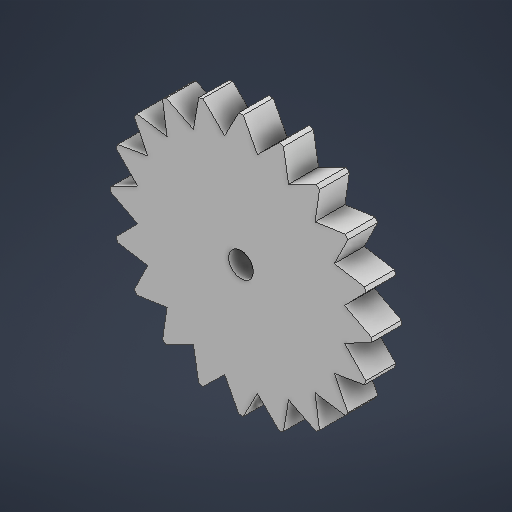
# Autodesk Inventor part: Gear_Basic
Saved by Autodesk Inventor 2026.1 (Build 301233020, 233B)
## iProperties
Created: 2026-03-11
Part Number: Gear_Basic
Material: Generic
Document SubType Name: Modeling
Designer: elaij
Density: 1 g/cm^3
Appearance: Default
Author: elaij
Autodesk Inventor part; units mm, degrees
ref_plane "YZ Plane" through (0, 0, 0) normal (1, 0, 0) x (0, 1, 0)
ref_plane "XZ Plane" through (0, 0, 0) normal (0, 1, 0) x (-1, 0, 0)
ref_plane "XY Plane" through (0, 0, 0) normal (0, 0, 1) x (1, 0, 0)
sketch "Sketch1" plane through (0, 0, 0) normal (0, 0, 1) x (1, 0, 0)
  circle A0 centre (0, 0) radius 22.5
  circle A1 centre (0, 0) radius 17.5
  line L0 (0, 0) -> (0, 22.5)
  line L1 (0, 22.5) -> (0, 0)
  line L2 (6.9529, 21.3988) -> (0, 0)
  line L3 (0, 0) -> (2.7376, 17.2845)
  line L4 (0, 22.5) -> (2.7376, 17.2845)
  line L5 (6.9529, 21.3988) -> (2.7376, 17.2845)
  line L6 (-6.9529, 21.3988) -> (-2.7376, 17.2845)
  line L7 (0, 22.5) -> (-2.7376, 17.2845)
  line L8 (-13.2252, 18.2029) -> (-7.9448, 15.5926)
  line L9 (-6.9529, 21.3988) -> (-7.9448, 15.5926)
  line L10 (-18.2029, 13.2252) -> (-12.3744, 12.3744)
  line L11 (-13.2252, 18.2029) -> (-12.3744, 12.3744)
  line L12 (-21.3988, 6.9529) -> (-15.5926, 7.9448)
  line L13 (-18.2029, 13.2252) -> (-15.5926, 7.9448)
  line L14 (-22.5, 0) -> (-17.2845, 2.7376)
  line L15 (-21.3988, 6.9529) -> (-17.2845, 2.7376)
  line L16 (-21.3988, -6.9529) -> (-17.2845, -2.7376)
  line L17 (-22.5, 0) -> (-17.2845, -2.7376)
  line L18 (-18.2029, -13.2252) -> (-15.5926, -7.9448)
  line L19 (-21.3988, -6.9529) -> (-15.5926, -7.9448)
  line L20 (-13.2252, -18.2029) -> (-12.3744, -12.3744)
  line L21 (-18.2029, -13.2252) -> (-12.3744, -12.3744)
  line L22 (-6.9529, -21.3988) -> (-7.9448, -15.5926)
  line L23 (-13.2252, -18.2029) -> (-7.9448, -15.5926)
  line L24 (0, -22.5) -> (-2.7376, -17.2845)
  line L25 (-6.9529, -21.3988) -> (-2.7376, -17.2845)
  line L26 (6.9529, -21.3988) -> (2.7376, -17.2845)
  line L27 (0, -22.5) -> (2.7376, -17.2845)
  line L28 (13.2252, -18.2029) -> (7.9448, -15.5926)
  line L29 (6.9529, -21.3988) -> (7.9448, -15.5926)
  line L30 (18.2029, -13.2252) -> (12.3744, -12.3744)
  line L31 (13.2252, -18.2029) -> (12.3744, -12.3744)
  line L32 (21.3988, -6.9529) -> (15.5926, -7.9448)
  line L33 (18.2029, -13.2252) -> (15.5926, -7.9448)
  line L34 (22.5, 0) -> (17.2845, -2.7376)
  line L35 (21.3988, -6.9529) -> (17.2845, -2.7376)
  line L36 (21.3988, 6.9529) -> (17.2845, 2.7376)
  line L37 (22.5, 0) -> (17.2845, 2.7376)
  line L38 (18.2029, 13.2252) -> (15.5926, 7.9448)
  line L39 (21.3988, 6.9529) -> (15.5926, 7.9448)
  line L40 (13.2252, 18.2029) -> (12.3744, 12.3744)
  line L41 (18.2029, 13.2252) -> (12.3744, 12.3744)
  line L42 (6.9529, 21.3988) -> (7.9448, 15.5926)
  line L43 (13.2252, 18.2029) -> (7.9448, 15.5926)
  point P0 (-22.5, 0)
  point P1 (-6.9529, -21.3988)
  point P2 (0, -22.5)
  point P3 (6.9529, -21.3988)
  point P4 (13.2252, -18.2029)
  point P5 (18.2029, -13.2252)
  point P6 (21.3988, -6.9529)
  point P7 (22.5, 0)
  point P8 (21.3988, 6.9529)
  point P9 (18.2029, 13.2252)
  point P10 (15.5926, 7.9448)
  point P11 (12.3744, 12.3744)
  point P12 (7.9448, 15.5926)
  point P13 (-21.3988, 6.9529)
  point P14 (-22.5, 0)
  point P15 (-21.3988, -6.9529)
  point P16 (-18.2029, -13.2252)
  point P17 (-13.2252, -18.2029)
  point P18 (-6.9529, -21.3988)
  point P19 (0, -22.5)
  point P20 (6.9529, -21.3988)
  point P21 (13.2252, -18.2029)
  point P22 (22.5, 0)
  point P23 (18.2029, 13.2252)
  point P24 (13.2252, 18.2029)
  dimension "d4" = 45
  dimension "d28" = 5
  dimension "d2" = 360
  dimension "d6" = 18
  dimension "d7" = 9
  dimension "d10" = 360
  dimension "d14" = 360
  constraints: 88 end point, 3 coincident, 1 collinear, 1 vertical, 1 vertical alignment, 148 other
  measures "d6" angle of L0 L2
  measures "d7" angle of L0 L3
extrude "Extrusion1" add sketch "Sketch1" along normal blind 5 contours L34 A1 L37 | L36 A1 L39 | L32 A1 L35 | A1 L0 L2 | L38 A1 L41 | L30 A1 L33 | L40 A1 L43 | L28 A1 L31 | L42 A1 L2 | L2 A1 L5 | L26 A1 L29 | L4 A1 L0 | L0 A1 L7 | L2 L3 A1 | L3 L0 A1 | L24 A1 L27 | L6 A1 L9 | L22 A1 L25 | L8 A1 L11 | L20 A1 L23 | L10 A1 L13 | L18 A1 L21 | L12 A1 L15 | L16 A1 L19 | L14 A1 L17
sketch "Sketch2" plane through (0, 0, 0) normal (0, 0, -1) x (-1, 0, 0)
  line L0 (-2.7376, 17.2845) -> (0, 22.5) projected
  circle A0 centre (0, 0) radius 22.5
  circle A1 centre (0, 0) radius 21.8
  dimension "d18" = 0.7
  constraints: 2 coincident, 1 centre point, 1 vertical alignment, 2 other
extrude "Extrusion2" cut sketch "Sketch2" against normal blind 5
sketch "Sketch3" plane through (0, 0, 0) normal (0, 0, -1) x (-1, 0, 0)
  point P0 (0, 0)
hole "Hole1" at (0, 0, 0) direction (0, 0, 1) diameter 4.134 depth 14.2 tip angle 118
body "Solid1"
